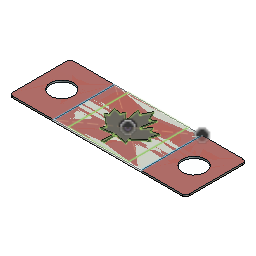
75x75mm Squat rack tubing (Autodesk Fusion 360 design; units mm, degrees)
Autodesk Fusion 360 part; units mm, degrees
sketch "Sketch1" plane through (0, 0, 0) normal (0, 0, 1) x (1, 0, 0)
  line L0 (225, 37.5) -> (-225, 37.5)
  line L1 (-225, 37.5) -> (-225, -37.5)
  line L2 (-225, -37.5) -> (225, -37.5)
  line L3 (225, -37.5) -> (225, 37.5)
  line L4 (225, 37.5) -> (-225, -37.5) construction
  line L5 (-225, 37.5) -> (225, -37.5) construction
  circle A0 centre (0, 2.4403) radius 13
  circle A1 centre (-200, 2.4403) radius 13
  circle A2 centre (-150, 2.4403) radius 13
  circle A3 centre (-100, 2.4403) radius 13
  circle A4 centre (-50, 2.4403) radius 13
  circle A5 centre (50, 2.4403) radius 13
  circle A6 centre (100, 2.4403) radius 13
  circle A7 centre (150, 2.4403) radius 13
  circle A8 centre (200, 2.4403) radius 13
  dimension "d6" = 450
  dimension "d7" = 75
  dimension "d8" = 26
  dimension "d11" = 50
  dimension "d12" = 0
  constraint horizontal L0
  constraint perpendicular L0 L1
  constraint parallel L0 L2
  constraint parallel L1 L3
  constraint coincident L4 origin
  constraint coincident L5 origin
  measures "d6" distance of L1.end L2.end
  measures "d7" distance of L0.end L1.end
  measures "d8" diameter of A0
extrude "Extrude1" add sketch "Sketch1" along normal blind 75 makes body 1
sketch "Sketch2" plane through (0, 37.5, 0) normal (0, 1, 0) x (-1, 0, 0)
  line L0 (-225, 0) -> (225, 0)
  line L1 (225, 0) -> (225, 75)
  line L2 (225, 75) -> (-225, 75)
  line L3 (-225, 75) -> (-225, 0)
  circle A0 centre (-175, 37.5) radius 13
  circle A1 centre (-125, 37.5) radius 13
  circle A2 centre (-75, 37.5) radius 13
  circle A3 centre (-25, 37.5) radius 13
  circle A4 centre (25, 37.5) radius 13
  circle A5 centre (75, 37.5) radius 13
  circle A6 centre (125, 37.5) radius 13
  circle A7 centre (175, 37.5) radius 13
  dimension "d15" = 26
  dimension "d16" = 37.5
  dimension "d17" = 50
  dimension "d20" = 50
  dimension "d21" = 0
  measures "d15" diameter of A0
  measures "d16" distance of L2 A0.centre
  measures "d17" distance of L3 A0.centre
extrude "Extrude2" cut sketch "Sketch2" against normal blind 75 contours A0 | A1 | A2 | A3 | A4 | A5 | A6 | A7 bodies 1
fillet "Fillet1" radius 2.5 4 edges at (0, 37.5, 75) (0, -37.5, 75) (0, -37.5, 0) (0, 37.5, 0) on bodies 1
ref_plane "WorkPlane1" through (0, 0, 76) normal (0, 0, 1) x (1, 0, 0)
sketch "Sketch3" plane through (0, 0, 76) normal (0, 0, 1) x (1, 0, 0)
  line L0 (100, -34.5) -> (-100, -34.5)
  line L1 (-100, -34.5) -> (-100, 34.5)
  line L2 (-100, 34.5) -> (100, 34.5)
  line L3 (100, 34.5) -> (100, -34.5)
  line L4 (100, -34.5) -> (-100, 34.5) construction
  line L5 (-100, -34.5) -> (100, 34.5) construction
  circle A0 centre (-75, 0) radius 13
  circle A1 centre (75, 0) radius 13
  dimension "d27" = 69
  dimension "d28" = 200
  dimension "d29" = 26
  dimension "d30" = 26
  dimension "d31" = 150
  dimension "d32" = 25
  constraint horizontal L0
  constraint perpendicular L0 L1
  constraint parallel L0 L2
  constraint parallel L1 L3
  constraint coincident L4 origin
  constraint coincident L5 origin
  measures "d27" distance of L0.end L1.end
  measures "d28" distance of L0.start L0.end
  measures "d29" diameter of A0
  measures "d30" diameter of A1
  measures "d31" distance of A0.centre A1.centre
  measures "d32" distance of L1 A0.centre
extrude "Extrude3" add sketch "Sketch3" along normal blind 2 separate body makes body 2
fillet "Fillet2" radius 4 4 edges at (100, 34.5, 77) (100, -34.5, 77) (-100, -34.5, 77) (-100, 34.5, 77) on bodies 2
sketch "Sketch4" plane through (0, 0, 78) normal (0, 0, 1) x (-1, 0, 0)
  circle A0 centre (-75, 0) radius 13
  circle A1 centre (75, 0) radius 13
  arc A2 (96, -34.5) -> (100, -30.5) centre (96, -30.5) ccw
  line L0 (100, -30.5) -> (100, 30.5)
  arc A3 (100, 30.5) -> (96, 34.5) centre (96, 30.5) ccw
  line L1 (96, 34.5) -> (-96, 34.5)
  arc A4 (-96, 34.5) -> (-100, 30.5) centre (-96, 30.5) ccw
  line L2 (-100, 30.5) -> (-100, -30.5)
  arc A5 (-100, -30.5) -> (-96, -34.5) centre (-96, -30.5) ccw
  line L3 (-96, -34.5) -> (96, -34.5)
  line L4 (34.0842, -34.6827) -> (-34.1783, -34.6827)
  line L5 (-34.1783, -34.6827) -> (-34.1783, 33.5798)
  line L6 (-34.1783, 33.5798) -> (34.0842, 33.5798)
  line L7 (34.0842, 33.5798) -> (34.0842, -34.6827)
  line L8 (-1.3271, 28.318) -> (-0.6871, 16.0448)
  spline S0 degree 3 poles (-0.6871, 16.0448) (-0.6778, 15.8429) (-0.7138, 15.6415) (-0.7926, 15.4555) knots 0 0 0 0 1 1 1 1
  spline S1 degree 3 poles (-0.7926, 15.4555) (-0.8715, 15.2695) (-0.9911, 15.1036) (-1.1424, 14.9698) knots 0 0 0 0 1 1 1 1
  spline S2 degree 3 poles (-1.1424, 14.9698) (-1.294, 14.8361) (-1.4734, 14.738) (-1.6679, 14.683) knots 0 0 0 0 1 1 1 1
  spline S3 degree 3 poles (-1.6679, 14.683) (-1.8621, 14.6277) (-2.0663, 14.6168) (-2.2656, 14.6512) knots 0 0 0 0 1 1 1 1
  line L9 (-2.2656, 14.6512) -> (-14.4816, 16.7986)
  line L10 (-14.4816, 16.7986) -> (-12.832, 12.2477)
  spline S4 degree 3 poles (-12.832, 12.2477) (-12.765, 12.0668) (-12.7566, 11.8691) (-12.8076, 11.6831) knots 0 0 0 0 1 1 1 1
  spline S5 degree 3 poles (-12.8076, 11.6831) (-12.8587, 11.4968) (-12.9666, 11.3312) (-13.1164, 11.2095) knots 0 0 0 0 1 1 1 1
  line L11 (-13.1164, 11.2095) -> (-26.4987, 0.373)
  line L12 (-26.4987, 0.373) -> (-23.4838, -1.0349)
  spline S6 degree 3 poles (-23.4838, -1.0349) (-23.2801, -1.1312) (-23.1187, -1.2984) (-23.0298, -1.5053) knots 0 0 0 0 1 1 1 1
  spline S7 degree 3 poles (-23.0298, -1.5053) (-22.9406, -1.7122) (-22.9303, -1.9445) (-23.0004, -2.1586) knots 0 0 0 0 1 1 1 1
  line L13 (-23.0004, -2.1586) -> (-25.6455, -10.2931)
  line L14 (-25.6455, -10.2931) -> (-17.9376, -8.6577)
  spline S8 degree 3 poles (-17.9376, -8.6577) (-17.7286, -8.6141) (-17.5111, -8.6441) (-17.3219, -8.7426) knots 0 0 0 0 1 1 1 1
  spline S9 degree 3 poles (-17.3219, -8.7426) (-17.1328, -8.8411) (-16.9835, -9.002) (-16.8994, -9.1981) knots 0 0 0 0 1 1 1 1
  line L15 (-16.8994, -9.1981) -> (-15.4061, -12.7107)
  line L16 (-15.4061, -12.7107) -> (-9.3905, -6.2543)
  spline S10 degree 3 poles (-9.3905, -6.2543) (-9.2529, -6.1091) (-9.072, -6.0125) (-8.8749, -5.9789) knots 0 0 0 0 1 1 1 1
  spline S11 degree 3 poles (-8.8749, -5.9789) (-8.678, -5.9453) (-8.4753, -5.9765) (-8.2973, -6.0681) knots 0 0 0 0 1 1 1 1
  spline S12 degree 3 poles (-8.2973, -6.0681) (-8.1195, -6.1593) (-7.9761, -6.3059) (-7.8885, -6.4856) knots 0 0 0 0 1 1 1 1
  spline S13 degree 3 poles (-7.8885, -6.4856) (-7.8009, -6.6652) (-7.7742, -6.8684) (-7.812, -7.0647) knots 0 0 0 0 1 1 1 1
  line L17 (-7.812, -7.0647) -> (-10.7132, -22.0257)
  line L18 (-10.7132, -22.0257) -> (-6.0626, -19.3379)
  spline S14 degree 3 poles (-6.0626, -19.3379) (-5.9536, -19.2739) (-5.8324, -19.233) (-5.7067, -19.2178) knots 0 0 0 0 1 1 1 1
  spline S15 degree 3 poles (-5.7067, -19.2178) (-5.5811, -19.2025) (-5.4535, -19.2132) (-5.3323, -19.2492) knots 0 0 0 0 1 1 1 1
  spline S16 degree 3 poles (-5.3323, -19.2492) (-5.2109, -19.2852) (-5.0985, -19.3457) (-5.0014, -19.427) knots 0 0 0 0 1 1 1 1
  spline S17 degree 3 poles (-5.0014, -19.427) (-4.9045, -19.5083) (-4.8251, -19.6087) (-4.7685, -19.7219) knots 0 0 0 0 1 1 1 1
  line L19 (-4.7685, -19.7219) -> (-0.047, -28.9942)
  line L20 (-0.047, -28.9942) -> (4.6745, -19.7219)
  spline S18 degree 3 poles (4.6745, -19.7219) (4.7311, -19.6087) (4.8105, -19.5083) (4.9073, -19.427) knots 0 0 0 0 1 1 1 1
  spline S19 degree 3 poles (4.9073, -19.427) (5.0044, -19.3457) (5.1168, -19.2852) (5.2383, -19.2492) knots 0 0 0 0 1 1 1 1
  spline S20 degree 3 poles (5.2383, -19.2492) (5.3595, -19.2132) (5.487, -19.2025) (5.6127, -19.2178) knots 0 0 0 0 1 1 1 1
  spline S21 degree 3 poles (5.6127, -19.2178) (5.7383, -19.233) (5.8595, -19.2739) (5.9685, -19.3379) knots 0 0 0 0 1 1 1 1
  line L21 (5.9685, -19.3379) -> (10.619, -22.0257)
  line L22 (10.619, -22.0257) -> (7.7178, -7.0647)
  spline S22 degree 3 poles (7.7178, -7.0647) (7.68, -6.8684) (7.707, -6.6652) (7.7945, -6.4856) knots 0 0 0 0 1 1 1 1
  spline S23 degree 3 poles (7.7945, -6.4856) (7.882, -6.3059) (8.0255, -6.1593) (8.2033, -6.0681) knots 0 0 0 0 1 1 1 1
  spline S24 degree 3 poles (8.2033, -6.0681) (8.3811, -5.9765) (8.5838, -5.9453) (8.7809, -5.9789) knots 0 0 0 0 1 1 1 1
  spline S25 degree 3 poles (8.7809, -5.9789) (8.978, -6.0125) (9.1589, -6.1091) (9.2964, -6.2543) knots 0 0 0 0 1 1 1 1
  line L23 (9.2964, -6.2543) -> (15.312, -12.7107)
  line L24 (15.312, -12.7107) -> (16.8053, -9.1981)
  spline S26 degree 3 poles (16.8053, -9.1981) (16.8894, -9.002) (17.0387, -8.8411) (17.2279, -8.7426) knots 0 0 0 0 1 1 1 1
  spline S27 degree 3 poles (17.2279, -8.7426) (17.4172, -8.6441) (17.6346, -8.6141) (17.8434, -8.6577) knots 0 0 0 0 1 1 1 1
  line L25 (17.8434, -8.6577) -> (25.5514, -10.2931)
  line L26 (25.5514, -10.2931) -> (22.9062, -2.1586)
  spline S28 degree 3 poles (22.9062, -2.1586) (22.8361, -1.9445) (22.8466, -1.7122) (22.9356, -1.5053) knots 0 0 0 0 1 1 1 1
  spline S29 degree 3 poles (22.9356, -1.5053) (23.0246, -1.2984) (23.1861, -1.1312) (23.3898, -1.0349) knots 0 0 0 0 1 1 1 1
  line L27 (23.3898, -1.0349) -> (26.4047, 0.373)
  line L28 (26.4047, 0.373) -> (13.0224, 11.2095)
  spline S30 degree 3 poles (13.0224, 11.2095) (12.8725, 11.3312) (12.7645, 11.4968) (12.7135, 11.6831) knots 0 0 0 0 1 1 1 1
  spline S31 degree 3 poles (12.7135, 11.6831) (12.6625, 11.8691) (12.671, 12.0668) (12.738, 12.2477) knots 0 0 0 0 1 1 1 1
  line L29 (12.738, 12.2477) -> (14.3876, 16.7986)
  line L30 (14.3876, 16.7986) -> (2.1715, 14.6512)
  spline S32 degree 3 poles (2.1715, 14.6512) (1.9723, 14.6168) (1.768, 14.6277) (1.5738, 14.683) knots 0 0 0 0 1 1 1 1
  spline S33 degree 3 poles (1.5738, 14.683) (1.3793, 14.738) (1.1997, 14.8361) (1.0483, 14.9698) knots 0 0 0 0 1 1 1 1
  spline S34 degree 3 poles (1.0483, 14.9698) (0.897, 15.1036) (0.7774, 15.2695) (0.6986, 15.4555) knots 0 0 0 0 1 1 1 1
  spline S35 degree 3 poles (0.6986, 15.4555) (0.6197, 15.6415) (0.5837, 15.8429) (0.593, 16.0448) knots 0 0 0 0 1 1 1 1
  line L31 (0.593, 16.0448) -> (1.2328, 28.318)
  line L32 (1.2328, 28.318) -> (-1.3271, 28.318)
  line L33 (-49.7163, -34.5) -> (49.7163, -34.5)
  line L34 (49.7163, -34.5) -> (49.7163, 34.5)
  line L35 (49.7163, 34.5) -> (-49.7163, 34.5)
  line L36 (-49.7163, 34.5) -> (-49.7163, -34.5)
  line L37 (-49.7163, -34.5) -> (49.7163, 34.5) construction
  line L38 (49.7163, -34.5) -> (-49.7163, 34.5) construction
  constraint horizontal L33
  constraint perpendicular L33 L34
  constraint parallel L33 L35
  constraint parallel L34 L36
  constraint coincident L37 origin
  constraint coincident L38 origin
  constraint coincident L3 L33.start
extrude "Extrude4" add sketch "Sketch4" against normal blind 2 separate body contours L1 L3 L5 L6 L7 L33 L34 L35 L36 | L3 L5 L6 L7 L33 makes body 3
extrude "Extrude5" add sketch "Sketch4" along normal blind 1 separate body contours L8 S0 S1 S2 S3 L9 L10 S4 S5 L11 L12 S6 S7 L13 L14 S8 S9 L15 L16 S10 S11 S12 S13 L17 L18 S14 S15 S16 S17 L19 L20 S18 S19 S20 S21 L21 L22 S22 S23 S24 S25 L23 L24 S26 S27 L25 L26 S28 S29 L27 L28 S30 S31 L29 L30 S32 S33 S34 S35 L31 L32 makes body 4
hidden bodies 1
equation "HoleSize = 26 mm"
equation "HoleSpacing = 50 mm"
equation "TubingSize = 75 mm"
equation "BadgeWidth = 4"
equation "HoleCount = 9"
equation "d6 = HoleCount * HoleSpacing"
equation "d7 = TubingSize"
equation "d8 = HoleSize"
equation "d9 = HoleCount"
equation "d11 = HoleSpacing"
equation "d13 = TubingSize"
equation "d15 = HoleSize"
equation "d16 = TubingSize / 2"
equation "d17 = HoleSpacing"
equation "d18 = HoleCount - 1"
equation "d20 = HoleSpacing"
equation "d27 = TubingSize - 6 mm"
equation "d28 = BadgeWidth * HoleSpacing"
equation "d29 = HoleSize"
equation "d30 = HoleSize"
equation "d31 = ( BadgeWidth - 1 ) * HoleSpacing"
equation "d32 = HoleSpacing / 2"
equation "BadgeThickness = 2 mm"
equation "d34 = BadgeThickness"
